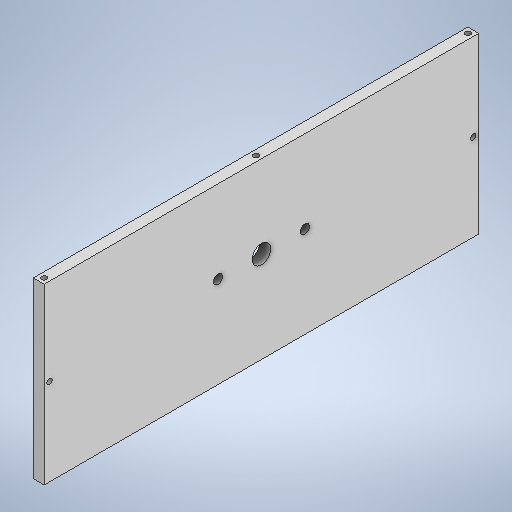
# Autodesk Inventor part: chassis_côté
Saved by Autodesk Inventor 2025.2 (Build 292293000, 293)
## iProperties
Created: 2026-03-16
Part Number: chassis_côté
Material: Générique
Document SubType Name: Modeling
Designer: genon
Density: 1 g/cm^3
Appearance: Par défaut
Author: genon
Autodesk Inventor part; units mm, degrees
ref_plane "YZ Plane" through (0, 0, 0) normal (1, 0, 0) x (0, 1, 0)
ref_plane "XZ Plane" through (0, 0, 0) normal (0, 1, 0) x (-1, 0, 0)
ref_plane "XY Plane" through (0, 0, 0) normal (0, 0, 1) x (1, 0, 0)
sketch "Esquisse1" plane through (0, 0, 0) normal (1, 0, 0) x (0, 1, 0)
  line L0 (0, 0) -> (80, 0)
  line L1 (80, 0) -> (80, -200)
  line L2 (80, -200) -> (0, -200)
  line L3 (0, -200) -> (0, 0)
  dimension "d0" = 80
  dimension "d1" = 200
  constraints: 8 end point, 2 parallel, 1 horizontal, 1 perpendicular
  measures "d0" distance of L1.end L2.end
  measures "d1" distance of L0.end L1.end
extrude "Extrusion1" add sketch "Esquisse1" along normal blind 5
sketch "Esquisse3" plane through (5, 0, 0) normal (1, 0, 0) x (0, 0, -1)
  line L0 (0, 0) -> (2.5, 0)
  line L1 (0, 0) -> (200, 0) projected
  line L2 (2.5, 0) -> (2.5, 40)
  line L3 (100, 0) -> (100, 21.0843)
  point P0 (2.5, 40)
  point P1 (197.5, 40)
  dimension "d15" = 2.5
  dimension "d16" = 40
  constraints: 6 end point, 1 coincident, 1 midpoint, 1 perpendicular, 1 point on line, 1 symmetric about line, 1 vertical
  measures "d15" distance of L0.start L0.end
  measures "d16" distance of L0.end L2.end
hole "Perçage2" at (5, 40, -2.5) at (5, 40, -197.5) direction (-1, 0, 0) diameter 2.459 end through all thread size "M3x0.5" class "6H" standard "ISO Metric profile"
sketch "Esquisse4" plane through (0, 0, -200) normal (0, -1, 0) x (1, 0, 0)
  line L0 (0, 200) -> (0, 197.5)
  line L1 (0, 0) -> (0, 200) projected
  line L2 (0, 197.5) -> (2.5, 197.5)
  line L3 (5, 200) -> (5, 0) projected
  point P0 (2.5, 2.5)
  point P1 (2.5, 100)
  dimension "d24" = 2.5
  dimension "d25" = 2.5
  dimension "d26" = 90
  constraints: 4 end point, 1 coincident, 1 perpendicular, 1 point on line
  measures "d24" distance of L0.start L0.end
  measures "d25" distance of L0.end L2.end
  measures "d26" angle of L2 L0
hole "Perçage3" at (2.5, 0, -2.5) at (2.5, 0, -197.5) at (2.5, 0, -100) direction (0, 1, 0) diameter 2.459 depth 8.8 tip angle 118 thread size "M3x0.5" class "6H" standard "ISO Metric profile"
sketch "Esquisse5" plane through (0, 80, 0) normal (0, 1, 0) x (1, 0, 0)
  line L0 (0, 0) -> (2.5, 0)
  line L1 (0, 0) -> (5, 0) projected
  line L2 (2.5, 0) -> (2.5, 2.5)
  line L3 (2.5, 0) -> (5, 0) construction
  line L4 (0, 200) -> (0, 0) projected
  line L5 (0, 100) -> (2.5, 100)
  point P0 (2.5, 197.5)
  dimension "d34" = 2.5
  dimension "d35" = 90
  constraints: 8 end point, 2 coincident, 2 horizontal, 2 midpoint, 2 perpendicular
  measures "d34" distance of L0.end L2.end
  measures "d35" angle of L3 L2
hole "Perçage4" at (2.5, 80, -2.5) at (2.5, 80, -197.5) at (2.5, 80, -100) direction (0, -1, 0) diameter 2.459 depth 8.8 tip angle 118 thread size "M3x0.5" class "6H" standard "ISO Metric profile"
sketch "Esquisse7" plane through (5, 0, 0) normal (1, 0, 0) x (0, 0, -1)
  line L0 (0, 0) -> (100, 0)
  line L1 (0, 0) -> (200, 0) projected
  line L2 (100, 0) -> (180, 0) construction
  line L3 (100, 80) -> (100, 10)
  line L4 (100, 80) -> (170, 80) construction
  line L5 (100, 10) -> (90.8075, 10)
  line L6 (100, 10) -> (80, 10)
  line L7 (80, 10) -> (80, 42)
  point P0 (120, 42)
  dimension "d50" = 100
  dimension "d53" = 70
  dimension "d54" = 90
  dimension "d67" = 20
  dimension "d68" = 32
  constraints: 14 end point, 3 horizontal, 2 perpendicular, 1 coincident, 1 midpoint, 1 point on line, 1 symmetric about line
  measures "d50" distance of L0.start L0.end
  measures "d53" distance of L3.start L3.end
  measures "d54" angle of L3 L4
  measures "d67" distance of L3.end L6.end
  measures "d68" distance of L6.end L7.end
hole "Perçage6" at (5, 42, -120) at (5, 42, -80) direction (-1, 0, 0) diameter 4.134 end through all thread size "M5x0.8" class "6H" standard "ISO Metric profile"
sketch "Esquisse8" plane through (5, 0, 0) normal (1, 0, 0) x (0, 0, -1)
  circle A0 centre (80, 42) radius 2.067 projected
  line L0 (80, 42) -> (100, 42)
  point P0 (0, 0)
  dimension "d69" = 20
  constraints: 2 end point, 1 coincident, 1 horizontal
  measures "d69" distance of L0.start L0.end
hole "Perçage7" at (5, 42, -100) direction (-1, 0, 0) diameter 8.5 end through all
